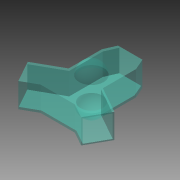
# Autodesk Inventor part: First try
Saved by Autodesk Inventor 2013 (Build 170138000, 138)
## iProperties
Created: 2014-03-26
Part Number: First try
Material: Agua
Document SubType Name: Chapa
Designer: Administrador
Density: 1 g/cm^3
Sheet Metal Rule: Por defecto_mm
Author: Administrador
Autodesk Inventor part; units mm, degrees
ref_plane "YZ Plane" through (0, 0, 0) normal (1, 0, 0) x (0, 1, 0)
ref_plane "XZ Plane" through (0, 0, 0) normal (0, 1, 0) x (-1, 0, 0)
ref_plane "XY Plane" through (0, 0, 0) normal (0, 0, 1) x (1, 0, 0)
sketch "Boceto3" plane through (0, 0, 0) normal (0, 0, 1) x (1, 0, 0)
  line L0 (0, 0) -> (0, 40) construction
  line L1 (0, 0) -> (30.537711, -17.101118) construction
  line L2 (0, 0) -> (-30.537711, -17.101118) construction
  line L3 (-10, 40) -> (10, 40)
  line L4 (25.651677, -25.826178) -> (35.423744, -8.376058)
  line L5 (-25.651677, -25.826178) -> (-35.423744, -8.376058)
  line L6 (-14, 30.698761) -> (14, 30.698761)
  line L7 (14, 30.698761) -> (14, -19.301239)
  line L8 (14, -19.301239) -> (-14, -19.301239)
  line L9 (-14, -19.301239) -> (-14, 30.698761)
  line L10 (14, 30.698761) -> (-14, -19.301239) construction
  line L11 (-14, 30.698761) -> (14, -19.301239) construction
  line L12 (-25.651677, -25.826178) -> (-14, -19.301239)
  line L13 (-10, 40) -> (-14, 30.698761)
  line L14 (10, 40) -> (14, 30.698761)
  line L15 (25.651677, -25.826178) -> (14, -19.301239)
  line L16 (35.423744, -8.376058) -> (14, 3.621239)
  line L17 (-35.423744, -8.376058) -> (-14, 3.621239)
  point P0 (0, 5.698761)
  dimension "d2" = 40
  dimension "d3" = 35
  dimension "d6" = 35
  dimension "d8" = 20
  dimension "d9" = 20
  dimension "d10" = 20
  dimension "d14" = 28
  dimension "d15" = 50
  constraints: 36 end point, 6 parallel, 5 perpendicular, 4 midpoint, 3 point on line, 1 coincident, 1 horizontal, 1 vertical
  measures "d2" distance of L0.start L0.end
  measures "d3" distance of L0.start L1.end
  measures "d6" distance of L0.start L2.end
  measures "d8" distance of L3.start L3.end
  measures "d9" distance of L4.start L4.end
  measures "d10" distance of L5.start L5.end
  measures "d14" distance of L7.end L8.end
  measures "d15" distance of L6.end L7.end
extrude "Extrusión1" add sketch "Boceto3" along normal blind 20
sketch "Boceto5" plane through (0, 0, 20) normal (0, 0, 1) x (1, 0, 0)
  circle A0 centre (0, 8.284973) radius 10
  line L0 (-10, 8.284973) -> (10, 8.284973)
  point P0 (0, 0)
  dimension "d21" = 20
  constraints: 2 end point, 2 point on circle, 1 centre point, 1 midpoint
  measures "d21" diameter of A0
revolve "Revolución2" add sketch "Boceto5" angle 360 about axis through (-10, 8.284973, 20) along (1, 0, 0) picked at (-1.893549, 5.541693) contours A0 L0
sketch "Boceto6" plane through (0, 0, 0) normal (0, 0, -1) x (-1, 0, 0)
  circle A0 centre (0, 8.284973) radius 10
  circle A1 centre (0, 8.284973) radius 10
  line L0 (4.608024, 17.16) -> (-4.608024, -0.590055)
  point P0 (0, 0)
  constraints: 2 end point, 2 point on circle, 1 centre point, 1 coincident, 1 midpoint, 3 other
revolve "Revolución3" add sketch "Boceto6" angle 360 about axis through (-4.608024, 17.16, 0) along (0.4608024, -0.8875027, 0) picked at (-3.310774, 8.672123) contours L0 A0
shell "Vaciado2" thickness 1 removed faces 3 at (3.333333, 40, 6.666667) at (-32.166388, -14.192765, 6.666667) at (28.909033, -20.009471, 6.666667)
equation "\"Radio_pliegue\" = Grosor"
equation "\"Anchura_desahogo_plegado\" = Grosor"
equation "\"Profundidad_desahogo_plegado\" = 0.5 * Grosor"
equation "\"Tamaño_destalonado\" = 4 * Grosor"
equation "\"Remanente_mínimo\" = 2 * Grosor"
equation "\"Radiodetransición\" = Radio_pliegue"
equation "\"Tamaño_de_radio_de_Jacobi\" = Radio_pliegue"
equation "\"TamañoSeparación\" = Grosor"
equation "\"d1\" = Radio_pliegue"
equation "\"Grosor\" = 0.5"
